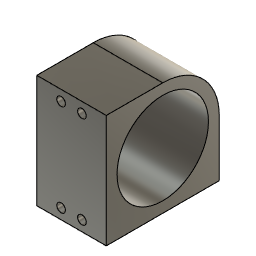
Version2EACCEnclsoure (Autodesk Fusion 360 archive; units mm, degrees)
design "Pipe Mount"
Autodesk Fusion 360 part; units mm, degrees
sketch "Sketch2" plane through (0, 0, 0) normal (1, 0, 0) x (0, 1, 0)
  circle A0 centre (0, 0) radius 16.7005
  circle A1 centre (0, 0) radius 20.6375
  line L0 (-20.6375, 20.6375) -> (20.6375, 20.6375)
  line L1 (20.6375, 20.6375) -> (20.6375, -20.6375)
  line L2 (20.6375, -20.6375) -> (-20.6375, -20.6375)
  line L3 (-20.6375, -20.6375) -> (-20.6375, 20.6375)
  line L4 (-20.6375, 20.6375) -> (0, 0) construction
  line L5 (0, 0) -> (-20.6375, -20.6375) construction
  line L6 (20.6375, -20.6375) -> (0, 0) construction
  line L7 (20.6375, 20.6375) -> (0, 0) construction
  line L8 (-20.6375, -20.6375) -> (-14.5929, -14.5929)
  line L9 (20.6375, -20.6375) -> (14.5929, -14.5929)
  dimension "d1" = 33.401
  dimension "d2" = 41.275
  dimension "d3" = 41.275
  constraint coincident A0.centre A1.centre
  constraint concentric A0 A1
  constraint horizontal L0
  constraint vertical L1
  constraint horizontal L2
  constraint vertical L3
  constraint perpendicular L4 L5
  constraint perpendicular L5 L6
  constraint perpendicular L4 L7
  constraint coincident A1 L8.end
  constraint coincident L5 L8.end
  constraint coincident L6 L9.end
  constraint coincident A1 L9.end
  measures "d1" diameter of A0
  measures "d2" diameter of A1
  measures "d3" distance of L0.start L0.end
extrude "Extrude1" add sketch "Sketch2" along normal blind 25.4 contours A1 | A1 L2 L9 | A1 L1 L9 | A1 L2 L8 | A1 L0 L3 | A1 L3 L8
sketch "Sketch3" plane through (0, 0, -20.6375) normal (0, 0, -1) x (1, 0, 0)
  line L0 (0, 20.6375) -> (0, -20.6375)
  line L1 (0, -20.6375) -> (25.4, -20.6375)
  line L2 (25.4, -20.6375) -> (25.4, 20.6375)
  line L3 (25.4, 20.6375) -> (0, 20.6375)
  line L4 (0, 16.8275) -> (25.4, 16.8275) construction
  line L5 (0, -16.8275) -> (25.4, -16.8275) construction
  circle A0 centre (3.81, 16.8275) radius 1.5875
  circle A1 centre (21.59, 16.8275) radius 1.5875
  circle A2 centre (3.81, -16.8275) radius 1.5875
  circle A3 centre (21.59, -16.8275) radius 1.5875
  dimension "d6" = 3.81
  dimension "d7" = 3.81
  dimension "d8" = 3.175
  dimension "d9" = 3.81
  dimension "d10" = 3.81
  dimension "d11" = 3.81
  dimension "d12" = 3.81
  constraint coincident L0 L4.start
  constraint coincident L2 L4.end
  constraint perpendicular L2 L4
  constraint coincident L0 L5.start
  constraint coincident L2 L5.end
  constraint perpendicular L2 L5
  constraint coincident L4 A0.centre
  constraint coincident L4 A1.centre
  constraint coincident L5 A2.centre
  constraint coincident L5 A3.centre
  constraint equal A2 A3
  constraint equal A1 A3
  constraint equal A0 A1
  measures "d6" distance of L3 L4
  measures "d7" distance of L1 L5
  measures "d8" diameter of A0
  measures "d9" distance of L4.start A0.centre
  measures "d10" distance of L4.end A1.centre
  measures "d11" horizontal distance of L0.end A2.centre
  measures "d12" distance of L5.end A3.centre
extrude "Extrude2" cut sketch "Sketch3" against normal blind 12.7 contours A0 | A1 | A2 | A3
sketch "Sketch4" plane through (0, -20.6375, 0) normal (0, -1, 0) x (1, 0, 0)
  line L0 (0, 20.6375) -> (0, -20.6375)
  line L1 (0, -20.6375) -> (25.4, -20.6375)
  line L2 (25.4, -20.6375) -> (25.4, 20.6375)
  line L3 (25.4, 20.6375) -> (0, 20.6375)
  line L4 (0, 16.8275) -> (25.4, 16.8275) construction
  line L5 (25.4, 16.8275) -> (25.4, -16.8275) construction
  line L6 (25.4, -16.8275) -> (0, -16.8275) construction
  line L7 (0, -16.8275) -> (0, 16.8275) construction
  line L8 (0, -20.6375) -> (25.4, -20.6375)
  circle A0 centre (8.89, 16.8275) radius 1.5875
  circle A1 centre (16.51, 16.8275) radius 1.5875
  circle A2 centre (8.89, -16.8275) radius 1.5875
  circle A3 centre (16.51, -16.8275) radius 1.5875
  dimension "d15" = 3.81
  dimension "d16" = 3.81
  dimension "d17" = 3.175
  dimension "d18" = 8.89
  dimension "d19" = 8.89
  dimension "d20" = 8.89
  dimension "d21" = 8.89
  constraint horizontal L4
  constraint vertical L5
  constraint horizontal L6
  constraint vertical L7
  constraint coincident L2 L5.end
  constraint coincident L0 L4.start
  constraint coincident L4 A0.centre
  constraint coincident L4 A1.centre
  constraint coincident L6 A2.centre
  constraint coincident L6 A3.centre
  constraint equal A0 A1
  constraint equal A1 A2
  constraint equal A2 A3
  measures "d15" distance of L6 L8
  measures "d16" distance of L3 L4
  measures "d17" diameter of A0
  measures "d18" distance of L4.start A0.centre
  measures "d19" distance of L4.end A1.centre
  measures "d20" distance of L6.end A2.centre
  measures "d21" distance of L5.end A3.centre
extrude "Extrude3" cut sketch "Sketch4" against normal blind 12.7 contours A0 | A1 | A2 | A3
equation "d7 = d6"
equation "d8 = ( 1 / 8 ) * 1 in"
equation "d10 = d9"
equation "d11 = d9"
equation "d12 = d9"
equation "d16 = d15"
equation "d19 = d18"
equation "d20 = d18"
equation "d21 = d20"
